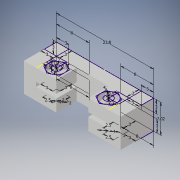
# Autodesk Inventor part: lidar_mount
Saved by Autodesk Inventor 2018 (Build 220112000, 112)
## iProperties
Created: 2018-04-30
Part Number: lidar_mount
Material: Generic
Document SubType Name: Modeling
Designer: dvyen
Density: 1 g/cm^3
Appearance: Default
Mass: 0.902142 g
Surface Area: 10.191 cm^2
Volume: 0.902142 cm^3
Author: dvyen
Autodesk Inventor part; units mm, degrees
ref_plane "YZ Plane" through (0, 0, 0) normal (1, 0, 0) x (0, 1, 0)
ref_plane "XZ Plane" through (0, 0, 0) normal (0, 1, 0) x (-1, 0, 0)
ref_plane "XY Plane" through (0, 0, 0) normal (0, 0, 1) x (1, 0, 0)
sketch "Sketch1" plane through (0, 0, 0) normal (0, 0, 1) x (1, 0, 0)
  line L0 (-11.9, 3.51) -> (11.9, 3.51)
  line L1 (11.9, 3.51) -> (11.9, -3.51)
  line L2 (11.9, -3.51) -> (-11.9, -3.51)
  line L3 (-11.9, -3.51) -> (-11.9, 3.51)
  line L4 (-11.9, 3.51) -> (11.9, -3.51) construction
  line L5 (11.9, 3.51) -> (-11.9, -3.51) construction
  line L6 (-11.9, 3.51) -> (-3.9, 3.51)
  line L7 (-3.9, 3.51) -> (-3.9, 0.51)
  line L8 (-3.9, 0.51) -> (-11.9, 0.51)
  line L9 (-11.9, 0.51) -> (-11.9, 3.51)
  line L10 (11.9, 3.51) -> (3.9, 3.51)
  line L11 (3.9, 3.51) -> (3.9, 0.51)
  line L12 (3.9, 0.51) -> (11.9, 0.51)
  line L13 (11.9, 0.51) -> (11.9, 3.51)
  line L14 (-11.9, -3.51) -> (-3.9, -3.51)
  line L15 (-3.9, -3.51) -> (-3.9, -0.51)
  line L16 (-3.9, -0.51) -> (-11.9, -0.51)
  line L17 (-11.9, -0.51) -> (-11.9, -3.51)
  line L18 (11.9, -3.51) -> (3.9, -3.51)
  line L19 (3.9, -3.51) -> (3.9, -0.51)
  line L20 (3.9, -0.51) -> (11.9, -0.51)
  line L21 (11.9, -0.51) -> (11.9, -3.51)
  line L22 (-11.9, 0.51) -> (-8.9, 0.51)
  line L23 (-8.9, 0.51) -> (-8.9, -0.51)
  line L24 (-8.9, -0.51) -> (-11.9, -0.51)
  line L25 (-11.9, -0.51) -> (-11.9, 0.51)
  line L26 (11.9, 0.51) -> (8.9, 0.51)
  line L27 (8.9, 0.51) -> (8.9, -0.51)
  line L28 (8.9, -0.51) -> (11.9, -0.51)
  line L29 (11.9, -0.51) -> (11.9, 0.51)
  point P0 (0, 0)
  dimension "d0" = 23.8
  dimension "d1" = 7.02
  dimension "d2" = 8
  dimension "d3" = 3
  dimension "d4" = 8
  dimension "d5" = 3
  dimension "d6" = 8
  dimension "d7" = 3
  dimension "d8" = 8
  dimension "d9" = 3
  dimension "d10" = 3
  dimension "d11" = 3
  constraints: 60 end point, 14 parallel, 7 horizontal, 7 perpendicular, 2 midpoint, 2 point on line
  measures "d0" distance of L1.end L2.end
  measures "d1" distance of L0.end L1.end
  measures "d2" distance of L7.end L8.end
  measures "d3" distance of L6.end L7.end
  measures "d4" distance of L12.end L11.end
  measures "d5" distance of L11.end L10.end
  measures "d6" distance of L16.end L15.end
  measures "d7" distance of L15.end L14.end
  measures "d8" distance of L19.end L20.end
  measures "d9" distance of L18.end L19.end
  measures "d10" distance of L23.end L24.end
  measures "d11" distance of L28.end L27.end
extrude "Extrusion1" add sketch "Sketch1" along normal blind 3 contours L0 L11 L12 L27 L20 L19 L2 L15 L16 L23 L8 L7
extrude "Extrusion2" add sketch "Sketch1" along normal blind 8 contours L0 L7 L8 L3 | L8 L23 L16 L3 | L0 L1 L12 L11 | L16 L15 L2 L3 | L1 L20 L27 L12 | L1 L2 L19 L20
sketch "Sketch5" plane through (-11.9, -3.51, 0) normal (0, -1, 0) x (1, 0, 0)
  line L0 (23.8, 0) -> (0, 0) projected
  line L1 (0, 0) -> (3, 0)
  line L2 (3, 0) -> (3, 3)
  line L3 (3, 3) -> (0, 3)
  line L4 (0, 3) -> (0, 0)
  line L5 (3, 3) -> (5.5, 3)
  line L6 (5.5, 3) -> (5.5, 5.5)
  line L7 (5.5, 5.5) -> (3, 5.5)
  line L8 (3, 5.5) -> (3, 3)
  circle A0 centre (5.5, 5.5) radius 1
  circle A1 centre (5.5, 5.5) radius 2
  line L9 (23.8, 0) -> (20.8, 0)
  line L10 (20.8, 0) -> (20.8, 3)
  line L11 (20.8, 3) -> (23.8, 3)
  line L12 (23.8, 3) -> (23.8, 0)
  line L13 (20.8, 3) -> (18.3, 3)
  line L14 (18.3, 3) -> (18.3, 5.5)
  line L15 (18.3, 5.5) -> (20.8, 5.5)
  line L16 (20.8, 5.5) -> (20.8, 3)
  circle A2 centre (18.3, 5.5) radius 1
  circle A3 centre (18.3, 5.5) radius 2
  point P0 (11.9, 0)
  dimension "d54" = 3
  dimension "d55" = 3
  dimension "d56" = 2.5
  dimension "d57" = 2.5
  dimension "d58" = 2
  dimension "d59" = 4
  dimension "d60" = 3
  dimension "d61" = 3
  dimension "d62" = 2.5
  dimension "d63" = 2.5
  dimension "d64" = 2
  dimension "d65" = 4
  constraints: 32 end point, 8 parallel, 4 centre point, 4 coincident, 4 horizontal, 4 perpendicular
  measures "d54" distance of L3.end L2.end
  measures "d55" distance of L2.end L1.end
  measures "d56" distance of L7.end L6.end
  measures "d57" distance of L6.end L5.end
  measures "d58" diameter of A0
  measures "d59" diameter of A1
  measures "d60" distance of L10.end L11.end
  measures "d61" distance of L9.end L10.end
  measures "d62" distance of L14.end L15.end
  measures "d63" distance of L13.end L14.end
  measures "d64" diameter of A2
  measures "d65" diameter of A3
extrude "Extrusion3" cut sketch "Sketch5" against normal blind 3 contours A0 L7 L6 | L6 L7 A0
extrude "Extrusion4" cut sketch "Sketch5" against normal blind 1.6 contours A3 L15 A2 L14 | L14 A2 L15 A3 | A1 L7 A0 L6 | L6 A0 L7 A1
extrude "Extrusion5" cut sketch "Sketch5" against normal blind 3 contours A2 L15 L14 | L14 L15 A2
sketch "Sketch6" plane through (-11.9, 3.51, 0) normal (0, 1, 0) x (1, 0, 0)
  line L0 (0, 0) -> (23.8, 0) projected
  line L1 (23.8, 0) -> (20.8, 0)
  line L2 (20.8, 0) -> (20.8, -3)
  line L3 (20.8, -3) -> (23.8, -3)
  line L4 (23.8, -3) -> (23.8, 0)
  line L5 (20.8, -3) -> (20.8, -8) projected
  line L6 (20.8, -3) -> (18.3, -3)
  line L7 (18.3, -3) -> (18.3, -5.5)
  line L8 (18.3, -5.5) -> (20.8, -5.5)
  line L9 (20.8, -5.5) -> (20.8, -3)
  circle A0 centre (18.3, -5.5) radius 1
  circle A1 centre (18.3, -5.5) radius 2
  circle A2 centre (18.3, -5.5) radius 2 projected
  line L10 (20.3, -6.6547) -> (18.3, -7.8094)
  line L11 (18.3, -7.8094) -> (16.3, -6.6547)
  line L12 (16.3, -6.6547) -> (16.3, -4.3453)
  line L13 (16.3, -4.3453) -> (18.3, -3.1906)
  line L14 (18.3, -3.1906) -> (20.3, -4.3453)
  line L15 (20.3, -4.3453) -> (20.3, -6.6547)
  line L16 (0, 0) -> (3, 0)
  line L17 (3, 0) -> (3, -3)
  line L18 (3, -3) -> (0, -3)
  line L19 (0, -3) -> (0, 0)
  line L20 (3, -3) -> (3, -8) projected
  line L21 (3, -3) -> (5.5, -3)
  line L22 (5.5, -3) -> (5.5, -5.5)
  line L23 (5.5, -5.5) -> (3, -5.5)
  line L24 (3, -5.5) -> (3, -3)
  circle A3 centre (5.5, -5.5) radius 1
  circle A4 centre (5.5, -5.5) radius 2
  circle A5 centre (5.5, -5.5) radius 2 projected
  line L25 (3.5, -4.3453) -> (5.5, -3.1906)
  line L26 (5.5, -3.1906) -> (7.5, -4.3453)
  line L27 (7.5, -4.3453) -> (7.5, -6.6547)
  line L28 (7.5, -6.6547) -> (5.5, -7.8094)
  line L29 (5.5, -7.8094) -> (3.5, -6.6547)
  line L30 (3.5, -6.6547) -> (3.5, -4.3453)
  point P0 (11.9, 0)
  point P1 (20.3, -5.5)
  point P2 (3.5, -5.5)
  dimension "d72" = 3
  dimension "d73" = 3
  dimension "d74" = 2.5
  dimension "d75" = 2.5
  dimension "d76" = 2
  dimension "d77" = 4
  dimension "d78" = 3
  dimension "d79" = 3
  dimension "d80" = 2.5
  dimension "d81" = 2.5
  dimension "d82" = 2
  dimension "d83" = 4
  constraints: 56 end point, 8 parallel, 6 coincident, 4 centre point, 4 horizontal, 4 perpendicular, 2 horizontal alignment, 2 midpoint, 2 point on line, 28 other
  measures "d72" distance of L3.end L2.end
  measures "d73" distance of L2.end L1.end
  measures "d74" distance of L8.end L7.end
  measures "d75" distance of L7.end L6.end
  measures "d76" diameter of A0
  measures "d77" diameter of A1
  measures "d78" distance of L17.end L18.end
  measures "d79" distance of L16.end L17.end
  measures "d80" distance of L22.end L23.end
  measures "d81" distance of L21.end L22.end
  measures "d82" diameter of A3
  measures "d83" diameter of A4
extrude "Extrusion6" cut sketch "Sketch6" against normal blind 1.6 contours A1 L7 A0 L8 | L8 A0 L7 A1 | L15 L10 A1 | A1 L14 L15 | L14 A1 L7 | L7 A1 L13 | L10 L11 A1 | A1 L12 L13 | L11 L12 A1
extrude "Extrusion7" cut sketch "Sketch6" against normal blind 3 contours A0 L7 L8 | L8 L7 A0
extrude "Extrusion8" cut sketch "Sketch6" against normal blind 3 contours A3 L22 L23 | L23 L22 A3
extrude "Extrusion9" cut sketch "Sketch6" against normal blind 1.6 contours A4 L22 A3 L23 | L30 L25 A4 | L23 A3 L22 A4 | A4 L29 L30 | L26 A4 L22 | L22 A4 L25 | A4 L28 L29 | L26 L27 A4 | A4 L27 L28
extrude "Extrusion10" cut sketch "Sketch5" against normal blind 2 contours A1 L7 A0 L6 | L6 A0 L7 A1
extrude "Extrusion11" cut sketch "Sketch5" against normal blind 2 contours A3 L15 A2 L14 | L14 A2 L15 A3
body "Solid1"
